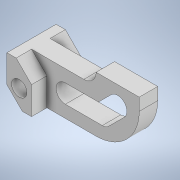
# Autodesk Inventor part: 1번부품
Saved by Autodesk Inventor 2022 (Build 260153000, 153)
## iProperties
Created: 2021-09-04
Part Number: 1번부품
Material: 일반
Document SubType Name: Modeling
Designer: 서울공업고등학교
Density: 1 g/cm^3
Appearance: 기본값
Author: 서울공업고등학교
Autodesk Inventor part; units mm, degrees
ref_plane "YZ Plane" through (0, 0, 0) normal (1, 0, 0) x (0, 1, 0)
ref_plane "XZ Plane" through (0, 0, 0) normal (0, 1, 0) x (-1, 0, 0)
ref_plane "XY Plane" through (0, 0, 0) normal (0, 0, 1) x (1, 0, 0)
sketch "스케치1" plane through (0, 0, 0) normal (0, 0, 1) x (1, 0, 0)
  line L0 (0, 0) -> (0, -14)
  line L1 (0, -14) -> (38, -14)
  line L2 (38, -14) -> (38, 4)
  line L3 (38, 4) -> (24, 4)
  line L4 (24, 4) -> (24, 0)
  line L5 (24, 0) -> (0, 0)
  line L6 (8, 0) -> (8, -14)
  dimension "d0" = 18
  dimension "d1" = 38
  dimension "d2" = 14
  dimension "d3" = 14
  dimension "d4" = 8
  constraints: 14 end point, 4 perpendicular, 2 point on line, 2 vertical, 1 horizontal
  measures "d0" distance of L1.end L2.end
  measures "d1" distance of L0.end L1.end
  measures "d2" distance of L0.start L0.end
  measures "d3" distance of L2.end L3.end
  measures "d4" distance between parallel lines of L6 L0
extrude "돌출1" add sketch "스케치1" along normal mid plane 6 contours L5 L4 L3 L2 L1 L6
extrude "돌출2" add sketch "스케치1" along normal mid plane 16 contours L5 L6 L1 L0
fillet "모깎기1" radius 4 1 edges at (24, 0, 0)
fillet "모깎기2" radius 14 1 edges at (38, -14, 0)
chamfer "모따기1" distance 5 angle 45 1 edges at (0, -14, 0)
chamfer "모따기2" distance 5 angle 45 1 edges at (8, 0, 5.5)
chamfer "모따기3" distance 5 angle 45 1 edges at (8, 0, -5.5)
sketch "스케치2" plane through (0, 0, 8) normal (0, 0, 1) x (1, 0, 0)
  circle A0 centre (4, -8) radius 2.5
  line L0 (0, 0) -> (0, -9) projected
  line L1 (5, -14) -> (8, -14) projected
  dimension "d20" = 5
  dimension "d21" = 4
  dimension "d22" = 6
  constraints: 1 centre point
  measures "d20" diameter of A0
  measures "d21" distance from line of L0 A0.centre
  measures "d22" distance from line of A0.centre L1
sketch "스케치3" plane through (0, 0, 3) normal (0, 0, 1) x (1, 0, 0)
  line L0 (31, -2) -> (26, -7) construction
  line L1 (28.8787, 0.1213) -> (23.8787, -4.8787)
  line L2 (28.1213, -9.1213) -> (33.1213, -4.1213)
  arc A0 (33.1213, -4.1213) -> (28.8787, 0.1213) centre (31, -2) ccw
  arc A1 (23.8787, -4.8787) -> (28.1213, -9.1213) centre (26, -7) ccw
  line L3 (38, 0) -> (38, 4) projected
  line L4 (38, 4) -> (24, 4) projected
  line L5 (26, -7) -> (14, -7) construction
  line L6 (26, -4) -> (14, -4)
  line L7 (14, -10) -> (26, -10)
  arc A2 (26, -10) -> (26, -4) centre (26, -7) ccw
  arc A3 (14, -4) -> (14, -10) centre (14, -7) ccw
  point P0 (0, 0)
  point P1 (28.5, -4.5)
  point P2 (20, -7)
  point P3 (24.7574, -4)
  dimension "d23" = 6
  dimension "d24" = 45
  dimension "d25" = 7
  dimension "d26" = 6
  dimension "d27" = 6
  dimension "d28" = 24
  dimension "d29" = 5
  constraints: 16 end point, 8 point on circle, 8 tangent, 4 centre point, 2 midpoint, 2 parallel, 1 horizontal
  measures "d23" diameter of A1
  measures "d24" angle of L3 L0
  measures "d25" distance from line of L3 L0.start
  measures "d26" distance from line of L4 L0.start
  measures "d27" diameter of A3
  measures "d28" distance from line of L3 L5.end
  measures "d29" vertical distance of L5.end L0.start
extrude "돌출3" cut sketch "스케치3" against normal blind 16
extrude "돌출4" cut sketch "스케치2" against normal blind 16
sketch "스케치4" plane through (0, 0, -8) normal (-1, 0, 0) x (0, 0, 1)
  line L0 (3.7292, -1.2202) -> (13.2257, -1.2202) construction
  line L1 (13.2257, -1.2202) -> (13.2257, -8.3293) construction
  line L2 (13.2257, -8.3293) -> (3.7292, -8.3293) construction
  line L3 (3.7292, -8.3293) -> (3.7292, -1.2202) construction
  line L4 (7.936, -7.4487) -> (4.1741, -7.4487)
  line L5 (4.1741, -7.4487) -> (4.1741, -6.5837)
  spline S0 degree 2 poles (4.1741, -6.5837) (4.5795, -6.203) (5.3012, -5.4961) (5.6472, -5.1155) knots 0 0 0 1 2 2 2
  spline S1 degree 2 poles (5.6472, -5.1155) (6.3442, -4.3493) (6.8534, -3.4299) (6.8534, -2.9405) knots 0 0 0 1 2 2 2
  spline S2 degree 2 poles (6.8534, -2.9405) (6.8534, -2.6834) (6.6952, -2.2979) (6.5518, -2.1743) knots 0 0 0 1 2 2 2
  spline S3 degree 2 poles (6.5518, -2.1743) (6.4085, -2.0507) (6.0328, -1.9271) (5.8054, -1.9271) knots 0 0 0 1 2 2 2
  spline S4 degree 2 poles (5.8054, -1.9271) (5.5879, -1.9271) (5.143, -2.0359) (4.9403, -2.1199) knots 0 0 0 1 2 2 2
  spline S5 degree 2 poles (4.9403, -2.1199) (4.7673, -2.1891) (4.446, -2.3868) (4.3471, -2.456) knots 0 0 0 1 2 2 2
  line L6 (4.3471, -2.456) -> (4.3027, -2.456)
  line L7 (4.3027, -2.456) -> (4.3027, -1.586)
  spline S6 degree 2 poles (4.3027, -1.586) (4.5548, -1.4624) (5.4594, -1.2202) (5.8647, -1.2202) knots 0 0 0 1 2 2 2
  spline S7 degree 2 poles (5.8647, -1.2202) (6.7199, -1.2202) (7.6839, -2.1248) (7.6839, -2.896) knots 0 0 0 1 2 2 2
  spline S8 degree 2 poles (7.6839, -2.896) (7.6839, -3.2568) (7.5158, -3.8599) (7.3675, -4.117) knots 0 0 0 1 2 2 2
  spline S9 degree 2 poles (7.3675, -4.117) (7.2192, -4.3839) (6.7891, -4.9079) (6.5518, -5.16) knots 0 0 0 1 2 2 2
  spline S10 degree 2 poles (6.5518, -5.16) (6.1663, -5.5802) (5.2221, -6.4799) (4.9403, -6.7419) knots 0 0 0 1 2 2 2
  line L8 (4.9403, -6.7419) -> (7.936, -6.7419)
  line L9 (7.936, -6.7419) -> (7.936, -7.4487)
  line L10 (12.207, -7.4487) -> (9.2311, -7.4487)
  line L11 (9.2311, -7.4487) -> (9.2311, -6.8259)
  line L12 (9.2311, -6.8259) -> (10.3384, -6.8259)
  line L13 (10.3384, -6.8259) -> (10.3384, -2.7378)
  line L14 (10.3384, -2.7378) -> (9.2311, -2.7378)
  line L15 (9.2311, -2.7378) -> (9.2311, -2.1792)
  spline S11 degree 2 poles (9.2311, -2.1792) (9.8589, -2.1792) (10.4521, -1.8233) (10.4916, -1.329) knots 0 0 0 1 2 2 2
  line L16 (10.4916, -1.329) -> (11.1244, -1.329)
  line L17 (11.1244, -1.329) -> (11.1244, -6.8259)
  line L18 (11.1244, -6.8259) -> (12.207, -6.8259)
  line L19 (12.207, -6.8259) -> (12.207, -7.4487)
  point P0 (8, 0)
  constraints: 2 other
extrude "돌출5" cut sketch "스케치4" against normal blind 1
